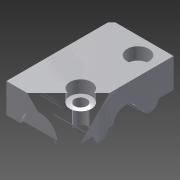
# Autodesk Inventor part: YAxisIdlerCap
Saved by Autodesk Inventor 2015 (Build 190159000, 159)
## iProperties
Created: 2014-08-08
Part Number: YAxisIdlerCap
Material: ABS Plastic
Document SubType Name: Modeling
Designer: t_clevj
Density: 1.06 g/cm^3
Appearance: Smooth - White
Author: t_clevj
Autodesk Inventor part; units mm, degrees
ref_plane "YZ Plane" through (0, 0, 0) normal (1, 0, 0) x (0, 1, 0)
ref_plane "XZ Plane" through (0, 0, 0) normal (0, 1, 0) x (-1, 0, 0)
ref_plane "XY Plane" through (0, 0, 0) normal (0, 0, 1) x (1, 0, 0)
sketch "Sketch1" plane through (0, 0, 0) normal (0, 0, 1) x (1, 0, 0)
  line L0 (0, 0) -> (20, 0)
  line L1 (20, 0) -> (20, 34)
  line L2 (20, 34) -> (0, 34)
  line L3 (0, 34) -> (0, 0)
  dimension "d0" = 20
  dimension "d1" = 34
  constraints: 8 end point, 2 parallel, 1 horizontal, 1 perpendicular
  measures "d0" distance of L1.end L2.end
  measures "d1" distance of L2.end L0.start
extrude "Extrusion1" add sketch "Sketch1" along normal blind 9.5
sketch "Sketch2" plane through (20, 0, 0) normal (1, 0, 0) x (0, 0, -1)
  line L0 (0, 0) -> (0, 34) projected
  circle A0 centre (0.5, 18.5) radius 4
  dimension "d4" = 8
  dimension "d11" = 0.5
  dimension "d26" = 18.5
  constraints: 1 centre point
  measures "d4" diameter of A0
  measures "d11" distance from line of L0 A0.centre
  measures "d26" vertical distance of L0.start A0.centre
extrude "Extrusion2" cut sketch "Sketch2" against normal up to next
sketch "Sketch3" plane through (0, 0, 9.5) normal (-1, 0, 0) x (0, 0, 1)
  line L0 (-9.5, 14.5314) -> (-9.5, 0) projected
  line L1 (-9.5, 34) -> (-9.5, 22.4686) projected
  circle A0 centre (-10, 6.5) radius 4.4
  circle A1 centre (-10, 28.5) radius 4.4
  arc A2 (-9.5, 14.5314) -> (-9.5, 22.4686) centre (-10, 18.5) ccw projected
  dimension "d7" = 8.8
  dimension "d8" = 8.8
  dimension "d9" = 0.5
  dimension "d10" = 0.5
  dimension "d64" = 10
  dimension "d65" = 12
  constraints: 2 centre point
  measures "d7" diameter of A0
  measures "d8" diameter of A1
  measures "d9" distance from line of L1 A1.centre
  measures "d10" distance from line of L0 A0.centre
  measures "d64" distance of A2.centre A1.centre
  measures "d65" distance of A2.centre A0.centre
extrude "Extrusion3" cut sketch "Sketch3" against normal blind 7
sketch "Sketch7" plane through (20, 0, 9.5) normal (1, 0, 0) x (0, 0, -1)
  line L0 (9.5, 22.4686) -> (9.5, 34) projected
  circle A0 centre (9.5, 28.5) radius 2.5
  line L1 (9.5, 2.1285) -> (9.5, 14.5314) projected
  circle A1 centre (9.5, 6.5) radius 2.5
  arc A2 (9.5, 22.4686) -> (9.5, 14.5314) centre (10, 18.5) ccw projected
  dimension "d33" = 5
  dimension "d34" = 5
  dimension "d61" = 10
  dimension "d62" = 12
  constraints: 2 centre point, 2 point on line
  measures "d33" diameter of A0
  measures "d34" diameter of A1
  measures "d61" vertical distance of A2.centre A0.centre
  measures "d62" vertical distance of A2.centre A1.centre
extrude "Extrusion7" add sketch "Sketch7" against normal up to surface (13 mm away)
sketch "Sketch8" plane through (0, 0, 9.5) normal (0, 0, 1) x (1, 0, 0)
  line L0 (20, 34) -> (0, 34) projected
  line L1 (0, 34) -> (0, 0) projected
  circle A0 centre (14, 28.5) radius 2
  circle A1 centre (14, 6.5314) radius 2
  line L2 (20, 22.4686) -> (20, 14.5314) projected
  line L3 (20, 22.4686) -> (0, 22.4686) projected
  line L4 (20, 14.5314) -> (20, 22.4686) projected
  line L5 (0, 14.5314) -> (20, 14.5314) projected
  line L6 (0, 22.4686) -> (0, 14.5314) projected
  dimension "d39" = 4
  dimension "d40" = 4
  dimension "d42" = 5.5
  dimension "d43" = 14
  dimension "d66" = 8
  constraints: 2 centre point, 1 vertical alignment
  measures "d39" diameter of A0
  measures "d40" diameter of A1
  measures "d42" distance from line of L0 A0.centre
  measures "d43" distance from line of L1 A0.centre
  measures "d66" distance from line of L5 A1.centre
extrude "Extrusion8" cut sketch "Sketch8" against normal up to next contours A0 | A1
sketch "Sketch9" plane through (0, 34, 0) normal (0, 1, 0) x (1, 0, 0)
  line L0 (20, 0) -> (0, 0) projected
  line L1 (20, 0) -> (20, -9.5) projected
  circle A0 centre (10, 0) radius 1.6
  dimension "d48" = 3.2
  dimension "d49" = 10
  constraints: 1 centre point, 1 midpoint
  measures "d48" diameter of A0
  measures "d49" distance from line of L1 A0.centre
extrude "Extrusion9" add sketch "Sketch9" against normal blind 6
sketch "Sketch10" plane through (0, 0, 9.5) normal (0, 0, 1) x (1, 0, 0)
  circle A0 centre (14, 28.5) radius 2 projected
  circle A1 centre (14, 6.5314) radius 2 projected
  circle A2 centre (14, 28.5) radius 3.5
  circle A3 centre (14, 6.5314) radius 3.5
  dimension "d52" = 7
  dimension "d53" = 7
  constraints: 2 centre point, 2 coincident
  measures "d52" diameter of A2
  measures "d53" diameter of A3
extrude "Extrusion10" cut sketch "Sketch10" against normal blind 4
sketch "Sketch11" plane through (0, 0, 0) normal (0, -1, 0) x (1, 0, 0)
  line L0 (0, 0) -> (20, 0) projected
  line L1 (0, 0) -> (0, 9.5) projected
  circle A0 centre (10, -0.5) radius 5.5
  dimension "d56" = 11
  dimension "d57" = 10
  dimension "d58" = 0.5
  constraints: 1 centre point
  measures "d56" diameter of A0
  measures "d57" distance from line of L1 A0.centre
  measures "d58" distance from line of L0 A0.centre
extrude "Extrusion11" cut sketch "Sketch11" against normal blind 1
body "Solid1"
